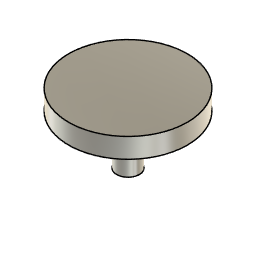
side_pulley_cap v2 (Autodesk Fusion 360 design; units mm, degrees)
Autodesk Fusion 360 part; units mm, degrees
sketch "Sketch1" plane through (0, 0, 0) normal (0, 1, 0) x (1, 0, 0)
  line L0 (0, 0) -> (1.15, 0)
  line L1 (1.15, 0) -> (1.15, -5)
  line L2 (1.15, -5) -> (6, -5)
  line L3 (6, -5) -> (6, -7)
  line L4 (6, -7) -> (0, -7)
  line L5 (0, -7) -> (0, 0)
  dimension "d1" = 1.15
  dimension "d2" = 5
  dimension "d5" = 6
  constraint coincident L0.start L5.end
  constraint horizontal L0
  constraint perpendicular L0 L1
  constraint perpendicular L1 L2
  constraint perpendicular L2 L3
  constraint perpendicular L3 L4
  constraint perpendicular L0 L5
  measures "d1" distance of L0.start L0.end
  measures "d2" distance of L0.end L1.end
  measures "d5" distance of L3.end L4.end
revolve "Revolve1" add sketch "Sketch1" angle 360 about axis through (0, 0, 7) along (0, 0, -1)
